minecraftdiamondsword for big CNC_v6 (Autodesk Fusion 360 design; units mm, degrees)
Autodesk Fusion 360 part; units mm, degrees
sketch "big huge diamond sword" plane through (0, 0, 0) normal (0, 0, 1) x (1, 0, 0)
  line L0 (-59.0146, -27.1837) -> (-49.7146, -27.1837)
  line L1 (-49.7146, -27.1837) -> (-49.7146, -17.8837)
  line L2 (-49.7146, -17.8837) -> (-59.0146, -17.8837)
  line L3 (-59.0146, -17.8837) -> (-59.0146, -27.1837)
  line L4 (-49.7146, -27.1837) -> (-40.4146, -27.1837)
  line L5 (-40.4146, -27.1837) -> (-40.4146, -17.8837)
  line L6 (-40.4146, -17.8837) -> (-49.7146, -17.8837)
  line L7 (-49.7146, -17.8837) -> (-49.7146, -27.1837)
  line L8 (-40.4146, -27.1837) -> (-31.1146, -27.1837)
  line L9 (-31.1146, -27.1837) -> (-31.1146, -17.8837)
  line L10 (-40.4146, -17.8837) -> (-40.4146, -27.1837)
  line L11 (-59.0146, -17.8837) -> (-49.7146, -17.8837)
  line L12 (-49.7146, -17.8837) -> (-49.7146, -8.5837)
  line L13 (-49.7146, -8.5837) -> (-59.0146, -8.5837)
  line L14 (-59.0146, -8.5837) -> (-59.0146, -17.8837)
  line L15 (-49.7146, -8.5837) -> (-40.4146, -8.5837)
  line L16 (-40.4146, -8.5837) -> (-40.4146, -17.8837)
  line L17 (-40.4146, -17.8837) -> (-49.7146, -17.8837)
  line L18 (-49.7146, -17.8837) -> (-49.7146, -8.5837)
  line L19 (-59.0146, -8.5837) -> (-49.7146, -8.5837)
  line L20 (-49.7146, -8.5837) -> (-49.7146, 0.7163)
  line L21 (-49.7146, 0.7163) -> (-59.0146, 0.7163)
  line L22 (-59.0146, 0.7163) -> (-59.0146, -8.5837)
  line L23 (-49.7146, -8.5837) -> (-40.4146, -8.5837)
  line L24 (-40.4146, -8.5837) -> (-40.4146, 0.7163)
  line L25 (-40.4146, 0.7163) -> (-49.7146, 0.7163)
  line L26 (-49.7146, 0.7163) -> (-49.7146, -8.5837)
  line L27 (-40.4146, -8.5837) -> (-31.1146, -8.5837)
  line L28 (-31.1146, -8.5837) -> (-31.1146, -17.8837)
  line L29 (-31.1146, -17.8837) -> (-40.4146, -17.8837)
  line L30 (-40.4146, -17.8837) -> (-40.4146, -8.5837)
  line L31 (-40.4146, -8.5837) -> (-31.1146, -8.5837)
  line L32 (-31.1146, -8.5837) -> (-31.1146, 0.7163)
  line L33 (-31.1146, 0.7163) -> (-40.4146, 0.7163)
  line L34 (-40.4146, 0.7163) -> (-40.4146, -8.5837)
  line L35 (-40.4146, 0.7163) -> (-31.1146, 0.7163)
  line L36 (-31.1146, 0.7163) -> (-31.1146, 10.0163)
  line L37 (-31.1146, 10.0163) -> (-40.4146, 10.0163)
  line L38 (-40.4146, 10.0163) -> (-40.4146, 0.7163)
  line L39 (-31.1146, 0.7163) -> (-21.8146, 0.7163)
  line L40 (-21.8146, 0.7163) -> (-21.8146, -8.5837)
  line L41 (-21.8146, -8.5837) -> (-31.1146, -8.5837)
  line L42 (-31.1146, -8.5837) -> (-31.1146, 0.7163)
  line L43 (-31.1146, 0.7163) -> (-21.8146, 0.7163)
  line L44 (-21.8146, 0.7163) -> (-21.8146, 10.0163)
  line L45 (-21.8146, 10.0163) -> (-31.1146, 10.0163)
  line L46 (-31.1146, 10.0163) -> (-31.1146, 0.7163)
  line L47 (-31.1146, 10.0163) -> (-21.8146, 10.0163)
  line L48 (-21.8146, 10.0163) -> (-21.8146, 19.3163)
  line L49 (-21.8146, 19.3163) -> (-31.1146, 19.3163)
  line L50 (-31.1146, 19.3163) -> (-31.1146, 10.0163)
  line L51 (-21.8146, 10.0163) -> (-12.5146, 10.0163)
  line L52 (-12.5146, 0.7163) -> (-21.8146, 0.7163)
  line L53 (-21.8146, 0.7163) -> (-21.8146, 10.0163)
  line L54 (-21.8146, 10.0163) -> (-12.5146, 10.0163)
  line L55 (-12.5146, 10.0163) -> (-12.5146, 19.3163)
  line L56 (-12.5146, 19.3163) -> (-21.8146, 19.3163)
  line L57 (-21.8146, 19.3163) -> (-21.8146, 10.0163)
  line L58 (-21.8146, 19.3163) -> (-12.5146, 19.3163)
  line L59 (-12.5146, 19.3163) -> (-12.5146, 28.6163)
  line L60 (-12.5146, 28.6163) -> (-21.8146, 28.6163)
  line L61 (-21.8146, 28.6163) -> (-21.8146, 19.3163)
  line L62 (-21.8146, 28.6163) -> (-31.1146, 28.6163)
  line L63 (-31.1146, 28.6163) -> (-31.1146, 37.9163)
  line L64 (-31.1146, 37.9163) -> (-21.8146, 37.9163)
  line L65 (-21.8146, 37.9163) -> (-21.8146, 28.6163)
  line L66 (-31.1146, 37.9163) -> (-21.8146, 37.9163)
  line L67 (-21.8146, 37.9163) -> (-21.8146, 47.2163)
  line L68 (-21.8146, 47.2163) -> (-31.1146, 47.2163)
  line L69 (-31.1146, 47.2163) -> (-31.1146, 37.9163)
  line L70 (-31.1146, 47.2163) -> (-40.4146, 47.2163)
  line L71 (-40.4146, 47.2163) -> (-40.4146, 56.5163)
  line L72 (-40.4146, 56.5163) -> (-31.1146, 56.5163)
  line L73 (-31.1146, 56.5163) -> (-31.1146, 47.2163)
  line L74 (-40.4146, 56.5163) -> (-31.1146, 56.5163)
  line L75 (-31.1146, 56.5163) -> (-31.1146, 65.8163)
  line L76 (-31.1146, 65.8163) -> (-40.4146, 65.8163)
  line L77 (-40.4146, 65.8163) -> (-40.4146, 56.5163)
  line L78 (-31.1146, 56.5163) -> (-21.8146, 56.5163)
  line L79 (-21.8146, 56.5163) -> (-21.8146, 65.8163)
  line L80 (-21.8146, 65.8163) -> (-31.1146, 65.8163)
  line L81 (-31.1146, 65.8163) -> (-31.1146, 56.5163)
  line L82 (-31.1146, 47.2163) -> (-21.8146, 47.2163)
  line L83 (-21.8146, 47.2163) -> (-21.8146, 56.5163)
  line L84 (-21.8146, 56.5163) -> (-31.1146, 56.5163)
  line L85 (-31.1146, 56.5163) -> (-31.1146, 47.2163)
  line L86 (-21.8146, 56.5163) -> (-12.5146, 56.5163)
  line L87 (-12.5146, 56.5163) -> (-12.5146, 47.2163)
  line L88 (-12.5146, 47.2163) -> (-21.8146, 47.2163)
  line L89 (-21.8146, 47.2163) -> (-21.8146, 56.5163)
  line L90 (-21.8146, 47.2163) -> (-12.5146, 47.2163)
  line L91 (-12.5146, 47.2163) -> (-12.5146, 37.9163)
  line L92 (-12.5146, 37.9163) -> (-21.8146, 37.9163)
  line L93 (-21.8146, 37.9163) -> (-21.8146, 47.2163)
  line L94 (-21.8146, 28.6163) -> (-12.5146, 28.6163)
  line L95 (-12.5146, 28.6163) -> (-12.5146, 37.9163)
  line L96 (-12.5146, 37.9163) -> (-21.8146, 37.9163)
  line L97 (-21.8146, 37.9163) -> (-21.8146, 28.6163)
  line L98 (-12.5146, 10.0163) -> (-3.2146, 10.0163)
  line L99 (-12.5146, 0.7163) -> (-12.5146, 10.0163)
  line L100 (-12.5146, 19.3163) -> (-3.2146, 19.3163)
  line L101 (-3.2146, 19.3163) -> (-3.2146, 10.0163)
  line L102 (-12.5146, 10.0163) -> (-12.5146, 19.3163)
  line L103 (-12.5146, 28.6163) -> (-3.2146, 28.6163)
  line L104 (-3.2146, 28.6163) -> (-3.2146, 19.3163)
  line L105 (-3.2146, 19.3163) -> (-12.5146, 19.3163)
  line L106 (-12.5146, 19.3163) -> (-12.5146, 28.6163)
  line L107 (-3.2146, 10.0163) -> (6.0854, 10.0163)
  line L108 (6.0854, 10.0163) -> (6.0854, 0.7163)
  line L109 (6.0854, 0.7163) -> (-3.2146, 0.7163)
  line L110 (-3.2146, 0.7163) -> (-3.2146, 10.0163)
  line L111 (-3.2146, 10.0163) -> (6.0854, 10.0163)
  line L112 (6.0854, 10.0163) -> (6.0854, 19.3163)
  line L113 (6.0854, 19.3163) -> (-3.2146, 19.3163)
  line L114 (-3.2146, 19.3163) -> (-3.2146, 10.0163)
  line L115 (6.0854, 10.0163) -> (15.3854, 10.0163)
  line L116 (15.3854, 10.0163) -> (15.3854, 0.7163)
  line L117 (15.3854, 0.7163) -> (6.0854, 0.7163)
  line L118 (6.0854, 0.7163) -> (6.0854, 10.0163)
  line L119 (15.3854, 0.7163) -> (24.6854, 0.7163)
  line L120 (24.6854, 0.7163) -> (24.6854, 10.0163)
  line L121 (24.6854, 10.0163) -> (15.3854, 10.0163)
  line L122 (15.3854, 10.0163) -> (15.3854, 0.7163)
  line L123 (24.6854, 0.7163) -> (33.9854, 0.7163)
  line L124 (33.9854, 0.7163) -> (33.9854, 10.0163)
  line L125 (33.9854, 10.0163) -> (24.6854, 10.0163)
  line L126 (24.6854, 10.0163) -> (24.6854, 0.7163)
  line L127 (15.3854, 0.7163) -> (24.6854, 0.7163)
  line L128 (24.6854, 0.7163) -> (24.6854, -8.5837)
  line L129 (24.6854, -8.5837) -> (15.3854, -8.5837)
  line L130 (15.3854, -8.5837) -> (15.3854, 0.7163)
  line L131 (24.6854, 0.7163) -> (33.9854, 0.7163)
  line L132 (33.9854, 0.7163) -> (33.9854, -8.5837)
  line L133 (33.9854, -8.5837) -> (24.6854, -8.5837)
  line L134 (24.6854, -8.5837) -> (24.6854, 0.7163)
  line L135 (-12.5146, 37.9163) -> (-3.2146, 37.9163)
  line L136 (-3.2146, 37.9163) -> (-3.2146, 28.6163)
  line L137 (-3.2146, 28.6163) -> (-12.5146, 28.6163)
  line L138 (-12.5146, 28.6163) -> (-12.5146, 37.9163)
  line L139 (-3.2146, 28.6163) -> (6.0854, 28.6163)
  line L140 (6.0854, 28.6163) -> (6.0854, 19.3163)
  line L141 (6.0854, 19.3163) -> (-3.2146, 19.3163)
  line L142 (-3.2146, 19.3163) -> (-3.2146, 28.6163)
  line L143 (-12.5146, 47.2163) -> (-3.2146, 47.2163)
  line L144 (-3.2146, 47.2163) -> (-3.2146, 37.9163)
  line L145 (-3.2146, 37.9163) -> (-12.5146, 37.9163)
  line L146 (-12.5146, 37.9163) -> (-12.5146, 47.2163)
  line L147 (-3.2146, 37.9163) -> (6.0854, 37.9163)
  line L148 (6.0854, 37.9163) -> (6.0854, 28.6163)
  line L149 (6.0854, 28.6163) -> (-3.2146, 28.6163)
  line L150 (-3.2146, 28.6163) -> (-3.2146, 37.9163)
  line L151 (-3.2146, 47.2163) -> (6.0854, 47.2163)
  line L152 (6.0854, 47.2163) -> (6.0854, 37.9163)
  line L153 (6.0854, 37.9163) -> (-3.2146, 37.9163)
  line L154 (-3.2146, 37.9163) -> (-3.2146, 47.2163)
  line L155 (6.0854, 19.3163) -> (15.3854, 19.3163)
  line L156 (15.3854, 19.3163) -> (15.3854, 10.0163)
  line L157 (15.3854, 10.0163) -> (6.0854, 10.0163)
  line L158 (6.0854, 10.0163) -> (6.0854, 19.3163)
  line L159 (15.3854, 19.3163) -> (24.6854, 19.3163)
  line L160 (24.6854, 19.3163) -> (24.6854, 10.0163)
  line L161 (24.6854, 10.0163) -> (15.3854, 10.0163)
  line L162 (15.3854, 10.0163) -> (15.3854, 19.3163)
  line L163 (6.0854, 28.6163) -> (15.3854, 28.6163)
  line L164 (15.3854, 28.6163) -> (15.3854, 19.3163)
  line L165 (15.3854, 19.3163) -> (6.0854, 19.3163)
  line L166 (6.0854, 19.3163) -> (6.0854, 28.6163)
  line L167 (6.0854, 37.9163) -> (15.3854, 37.9163)
  line L168 (15.3854, 37.9163) -> (15.3854, 28.6163)
  line L169 (15.3854, 28.6163) -> (6.0854, 28.6163)
  line L170 (6.0854, 28.6163) -> (6.0854, 37.9163)
  line L171 (15.3854, 28.6163) -> (6.0854, 28.6163)
  line L172 (6.0854, 28.6163) -> (6.0854, 37.9163)
  line L173 (6.0854, 37.9163) -> (15.3854, 37.9163)
  line L174 (15.3854, 37.9163) -> (15.3854, 28.6163)
  line L175 (15.3854, 28.6163) -> (24.6854, 28.6163)
  line L176 (24.6854, 28.6163) -> (24.6854, 37.9163)
  line L177 (24.6854, 37.9163) -> (15.3854, 37.9163)
  line L178 (15.3854, 37.9163) -> (15.3854, 28.6163)
  line L179 (6.0854, 37.9163) -> (15.3854, 37.9163)
  line L180 (15.3854, 37.9163) -> (15.3854, 47.2163)
  line L181 (15.3854, 47.2163) -> (6.0854, 47.2163)
  line L182 (6.0854, 47.2163) -> (6.0854, 37.9163)
  line L183 (15.3854, 37.9163) -> (24.6854, 37.9163)
  line L184 (24.6854, 37.9163) -> (24.6854, 47.2163)
  line L185 (24.6854, 47.2163) -> (15.3854, 47.2163)
  line L186 (15.3854, 47.2163) -> (15.3854, 37.9163)
  line L187 (24.6854, 37.9163) -> (33.9854, 37.9163)
  line L188 (33.9854, 37.9163) -> (33.9854, 47.2163)
  line L189 (33.9854, 47.2163) -> (24.6854, 47.2163)
  line L190 (24.6854, 47.2163) -> (24.6854, 37.9163)
  line L191 (-3.2146, 47.2163) -> (6.0854, 47.2163)
  line L192 (6.0854, 47.2163) -> (6.0854, 56.5163)
  line L193 (6.0854, 56.5163) -> (-3.2146, 56.5163)
  line L194 (-3.2146, 56.5163) -> (-3.2146, 47.2163)
  line L195 (6.0854, 47.2163) -> (15.3854, 47.2163)
  line L196 (15.3854, 47.2163) -> (15.3854, 56.5163)
  line L197 (15.3854, 56.5163) -> (6.0854, 56.5163)
  line L198 (6.0854, 56.5163) -> (6.0854, 47.2163)
  line L199 (15.3854, 56.5163) -> (6.0854, 56.5163)
  line L200 (6.0854, 56.5163) -> (6.0854, 65.8163)
  line L201 (6.0854, 65.8163) -> (15.3854, 65.8163)
  line L202 (15.3854, 65.8163) -> (15.3854, 56.5163)
  line L203 (15.3854, 47.2163) -> (24.6854, 47.2163)
  line L204 (24.6854, 47.2163) -> (24.6854, 56.5163)
  line L205 (24.6854, 56.5163) -> (15.3854, 56.5163)
  line L206 (15.3854, 56.5163) -> (15.3854, 47.2163)
  line L207 (15.3854, 56.5163) -> (24.6854, 56.5163)
  line L208 (24.6854, 56.5163) -> (24.6854, 65.8163)
  line L209 (24.6854, 65.8163) -> (15.3854, 65.8163)
  line L210 (15.3854, 65.8163) -> (15.3854, 56.5163)
  line L211 (24.6854, 47.2163) -> (33.9854, 47.2163)
  line L212 (33.9854, 47.2163) -> (33.9854, 56.5163)
  line L213 (33.9854, 56.5163) -> (24.6854, 56.5163)
  line L214 (24.6854, 56.5163) -> (24.6854, 47.2163)
  line L215 (15.3854, 65.8163) -> (24.6854, 65.8163)
  line L216 (24.6854, 65.8163) -> (24.6854, 75.1163)
  line L217 (24.6854, 75.1163) -> (15.3854, 75.1163)
  line L218 (15.3854, 75.1163) -> (15.3854, 65.8163)
  line L219 (33.9854, 47.2163) -> (43.2854, 47.2163)
  line L220 (43.2854, 47.2163) -> (43.2854, 56.5163)
  line L221 (43.2854, 56.5163) -> (33.9854, 56.5163)
  line L222 (33.9854, 56.5163) -> (33.9854, 47.2163)
  line L223 (24.6854, 56.5163) -> (33.9854, 56.5163)
  line L224 (33.9854, 56.5163) -> (33.9854, 65.8163)
  line L225 (33.9854, 65.8163) -> (24.6854, 65.8163)
  line L226 (24.6854, 65.8163) -> (24.6854, 56.5163)
  line L227 (33.9854, 65.8163) -> (43.2854, 65.8163)
  line L228 (43.2854, 65.8163) -> (43.2854, 75.1163)
  line L229 (43.2854, 75.1163) -> (33.9854, 75.1163)
  line L230 (33.9854, 75.1163) -> (33.9854, 65.8163)
  line L231 (33.9854, 65.8163) -> (24.6854, 65.8163)
  line L232 (24.6854, 65.8163) -> (24.6854, 75.1163)
  line L233 (24.6854, 75.1163) -> (33.9854, 75.1163)
  line L234 (33.9854, 75.1163) -> (33.9854, 65.8163)
  line L235 (33.9854, 65.8163) -> (43.2854, 65.8163)
  line L236 (43.2854, 65.8163) -> (43.2854, 56.5163)
  line L237 (43.2854, 56.5163) -> (33.9854, 56.5163)
  line L238 (33.9854, 56.5163) -> (33.9854, 65.8163)
  line L239 (24.6854, 75.1163) -> (33.9854, 75.1163)
  line L240 (33.9854, 75.1163) -> (33.9854, 84.4163)
  line L241 (33.9854, 84.4163) -> (24.6854, 84.4163)
  line L242 (24.6854, 84.4163) -> (24.6854, 75.1163)
  line L243 (33.9854, 75.1163) -> (43.2854, 75.1163)
  line L244 (43.2854, 75.1163) -> (43.2854, 84.4163)
  line L245 (43.2854, 84.4163) -> (33.9854, 84.4163)
  line L246 (33.9854, 84.4163) -> (33.9854, 75.1163)
  line L247 (43.2854, 56.5163) -> (52.5854, 56.5163)
  line L248 (52.5854, 56.5163) -> (52.5854, 65.8163)
  line L249 (52.5854, 65.8163) -> (43.2854, 65.8163)
  line L250 (43.2854, 65.8163) -> (43.2854, 56.5163)
  line L251 (43.2854, 65.8163) -> (52.5854, 65.8163)
  line L252 (52.5854, 65.8163) -> (52.5854, 75.1163)
  line L253 (52.5854, 75.1163) -> (43.2854, 75.1163)
  line L254 (43.2854, 75.1163) -> (43.2854, 65.8163)
  line L255 (43.2854, 75.1163) -> (52.5854, 75.1163)
  line L256 (52.5854, 75.1163) -> (52.5854, 84.4163)
  line L257 (52.5854, 84.4163) -> (43.2854, 84.4163)
  line L258 (43.2854, 84.4163) -> (43.2854, 75.1163)
  line L259 (33.9854, 84.4163) -> (43.2854, 84.4163)
  line L260 (43.2854, 84.4163) -> (43.2854, 93.7163)
  line L261 (43.2854, 93.7163) -> (33.9854, 93.7163)
  line L262 (33.9854, 93.7163) -> (33.9854, 84.4163)
  line L263 (52.5854, 65.8163) -> (61.8854, 65.8163)
  line L264 (61.8854, 65.8163) -> (61.8854, 75.1163)
  line L265 (61.8854, 75.1163) -> (52.5854, 75.1163)
  line L266 (52.5854, 75.1163) -> (52.5854, 65.8163)
  line L267 (43.2854, 84.4163) -> (52.5854, 84.4163)
  line L268 (52.5854, 84.4163) -> (52.5854, 93.7163)
  line L269 (52.5854, 93.7163) -> (43.2854, 93.7163)
  line L270 (43.2854, 93.7163) -> (43.2854, 84.4163)
  line L271 (52.5854, 75.1163) -> (61.8854, 75.1163)
  line L272 (61.8854, 75.1163) -> (61.8854, 84.4163)
  line L273 (61.8854, 84.4163) -> (52.5854, 84.4163)
  line L274 (52.5854, 84.4163) -> (52.5854, 75.1163)
  line L275 (52.5854, 84.4163) -> (61.8854, 84.4163)
  line L276 (61.8854, 84.4163) -> (61.8854, 93.7163)
  line L277 (61.8854, 93.7163) -> (52.5854, 93.7163)
  line L278 (52.5854, 93.7163) -> (52.5854, 84.4163)
  line L279 (61.8854, 75.1163) -> (71.1854, 75.1163)
  line L280 (71.1854, 75.1163) -> (71.1854, 84.4163)
  line L281 (71.1854, 84.4163) -> (61.8854, 84.4163)
  line L282 (61.8854, 84.4163) -> (61.8854, 75.1163)
  line L283 (43.2854, 93.7163) -> (52.5854, 93.7163)
  line L284 (52.5854, 93.7163) -> (52.5854, 103.0163)
  line L285 (52.5854, 103.0163) -> (43.2854, 103.0163)
  line L286 (43.2854, 103.0163) -> (43.2854, 93.7163)
  line L287 (61.8854, 93.7163) -> (71.1854, 93.7163)
  line L288 (71.1854, 93.7163) -> (71.1854, 84.4163)
  line L289 (71.1854, 84.4163) -> (61.8854, 84.4163)
  line L290 (61.8854, 84.4163) -> (61.8854, 93.7163)
  line L291 (52.5854, 93.7163) -> (61.8854, 93.7163)
  line L292 (61.8854, 93.7163) -> (61.8854, 103.0163)
  line L293 (61.8854, 103.0163) -> (52.5854, 103.0163)
  line L294 (52.5854, 103.0163) -> (52.5854, 93.7163)
  line L295 (61.8854, 93.7163) -> (71.1854, 93.7163)
  line L296 (71.1854, 93.7163) -> (71.1854, 103.0163)
  line L297 (71.1854, 103.0163) -> (61.8854, 103.0163)
  line L298 (61.8854, 103.0163) -> (61.8854, 93.7163)
  line L299 (71.1854, 84.4163) -> (80.4854, 84.4163)
  line L300 (80.4854, 84.4163) -> (80.4854, 93.7163)
  line L301 (80.4854, 93.7163) -> (71.1854, 93.7163)
  line L302 (71.1854, 93.7163) -> (71.1854, 84.4163)
  line L303 (52.5854, 103.0163) -> (61.8854, 103.0163)
  line L304 (61.8854, 103.0163) -> (61.8854, 112.3163)
  line L305 (61.8854, 112.3163) -> (52.5854, 112.3163)
  line L306 (52.5854, 112.3163) -> (52.5854, 103.0163)
  line L307 (61.8854, 112.3163) -> (71.1854, 112.3163)
  line L308 (71.1854, 112.3163) -> (71.1854, 103.0163)
  line L309 (71.1854, 103.0163) -> (61.8854, 103.0163)
  line L310 (61.8854, 103.0163) -> (61.8854, 112.3163)
  line L311 (71.1854, 93.7163) -> (80.4854, 93.7163)
  line L312 (80.4854, 93.7163) -> (80.4854, 103.0163)
  line L313 (80.4854, 103.0163) -> (71.1854, 103.0163)
  line L314 (71.1854, 103.0163) -> (71.1854, 93.7163)
  line L315 (71.1854, 103.0163) -> (80.4854, 103.0163)
  line L316 (80.4854, 103.0163) -> (80.4854, 112.3163)
  line L317 (80.4854, 112.3163) -> (71.1854, 112.3163)
  line L318 (71.1854, 112.3163) -> (71.1854, 103.0163)
  line L319 (61.8854, 112.3163) -> (71.1854, 112.3163)
  line L320 (71.1854, 112.3163) -> (71.1854, 121.6163)
  line L321 (71.1854, 121.6163) -> (61.8854, 121.6163)
  line L322 (61.8854, 121.6163) -> (61.8854, 112.3163)
  line L323 (71.1854, 112.3163) -> (80.4854, 112.3163)
  line L324 (80.4854, 112.3163) -> (80.4854, 121.6163)
  line L325 (80.4854, 121.6163) -> (71.1854, 121.6163)
  line L326 (71.1854, 121.6163) -> (71.1854, 112.3163)
  line L327 (80.4854, 93.7163) -> (89.7854, 93.7163)
  line L328 (89.7854, 93.7163) -> (89.7854, 103.0163)
  line L329 (89.7854, 103.0163) -> (80.4854, 103.0163)
  line L330 (80.4854, 103.0163) -> (80.4854, 93.7163)
  line L331 (80.4854, 103.0163) -> (89.7854, 103.0163)
  line L332 (89.7854, 103.0163) -> (89.7854, 112.3163)
  line L333 (89.7854, 112.3163) -> (80.4854, 112.3163)
  line L334 (80.4854, 112.3163) -> (80.4854, 103.0163)
  line L335 (80.4854, 112.3163) -> (71.1854, 112.3163)
  line L336 (71.1854, 112.3163) -> (71.1854, 121.6163)
  line L337 (71.1854, 121.6163) -> (80.4854, 121.6163)
  line L338 (80.4854, 121.6163) -> (80.4854, 112.3163)
  line L339 (80.4854, 112.3163) -> (89.7854, 112.3163)
  line L340 (89.7854, 112.3163) -> (89.7854, 121.6163)
  line L341 (89.7854, 121.6163) -> (80.4854, 121.6163)
  line L342 (80.4854, 121.6163) -> (80.4854, 112.3163)
  dimension "d249" = 9.3
  dimension "d250" = 9.3
  dimension "d251" = 9.3
  dimension "d252" = 9.3
  dimension "d253" = 9.3
  dimension "d254" = 9.3
  dimension "d255" = 9.3
  dimension "d256" = 9.3
  dimension "d261" = 9.3
  dimension "d262" = 9.3
  dimension "d263" = 9.3
  dimension "d264" = 9.3
  dimension "d265" = 9.3
  dimension "d266" = 9.3
  dimension "d267" = 9.3
  dimension "d268" = 9.3
  dimension "d271" = 9.3
  dimension "d272" = 9.3
  dimension "d273" = 9.3
  dimension "d274" = 9.3
  dimension "d275" = 9.3
  dimension "d276" = 9.3
  dimension "d277" = 9.3
  dimension "d278" = 9.3
  dimension "d279" = 9.3
  dimension "d280" = 9.3
  dimension "d281" = 9.3
  dimension "d282" = 9.3
  dimension "d283" = 9.3
  dimension "d284" = 9.3
  dimension "d285" = 9.3
  dimension "d286" = 9.3
  dimension "d287" = 9.3
  dimension "d288" = 9.3
  dimension "d289" = 9.3
  dimension "d290" = 9.3
  dimension "d291" = 9.3
  dimension "d292" = 9.3
  dimension "d293" = 9.3
  dimension "d294" = 9.3
  dimension "d295" = 9.3
  dimension "d296" = 9.3
  dimension "d297" = 9.3
  dimension "d298" = 9.3
  dimension "d299" = 9.3
  dimension "d300" = 9.3
  dimension "d301" = 9.3
  dimension "d302" = 9.3
  dimension "d303" = 9.3
  dimension "d304" = 9.3
  dimension "d309" = 9.3
  dimension "d310" = 9.3
  dimension "d311" = 9.3
  dimension "d312" = 9.3
  dimension "d313" = 9.3
  dimension "d314" = 9.3
  dimension "d315" = 9.3
  dimension "d316" = 9.3
  dimension "d319" = 9.3
  dimension "d320" = 9.3
  dimension "d321" = 9.3
  dimension "d322" = 9.3
  dimension "d323" = 9.3
  dimension "d324" = 9.3
  dimension "d325" = 9.3
  dimension "d326" = 9.3
  dimension "d327" = 9.3
  dimension "d328" = 9.3
  dimension "d329" = 9.3
  dimension "d330" = 9.3
  dimension "d331" = 9.3
  dimension "d332" = 9.3
  dimension "d333" = 9.3
  dimension "d334" = 9.3
  dimension "d335" = 9.3
  dimension "d336" = 9.3
  dimension "d337" = 9.3
  dimension "d338" = 9.3
  dimension "d339" = 9.3
  dimension "d340" = 9.3
  dimension "d341" = 9.3
  dimension "d342" = 9.3
  dimension "d343" = 9.3
  dimension "d344" = 9.3
  dimension "d345" = 9.3
  dimension "d346" = 9.3
  dimension "d347" = 9.3
  dimension "d348" = 9.3
  dimension "d349" = 9.3
  dimension "d350" = 9.3
  dimension "d351" = 9.3
  dimension "d352" = 9.3
  dimension "d353" = 9.3
  dimension "d354" = 9.3
  dimension "d355" = 9.3
  dimension "d356" = 9.3
  dimension "d357" = 9.3
  dimension "d358" = 9.3
  dimension "d359" = 9.3
  dimension "d360" = 9.3
  dimension "d361" = 9.3
  dimension "d362" = 9.3
  dimension "d363" = 9.3
  dimension "d364" = 9.3
  dimension "d365" = 9.3
  dimension "d366" = 9.3
  dimension "d367" = 9.3
  dimension "d368" = 9.3
  dimension "d369" = 9.3
  dimension "d370" = 9.3
  dimension "d371" = 9.3
  dimension "d372" = 9.3
  dimension "d373" = 9.3
  dimension "d374" = 9.3
  dimension "d375" = 9.3
  dimension "d376" = 9.3
  dimension "d377" = 9.3
  dimension "d378" = 9.3
  dimension "d379" = 9.3
  dimension "d380" = 9.3
  dimension "d381" = 9.3
  dimension "d382" = 9.3
  dimension "d383" = 9.3
  dimension "d384" = 9.3
  dimension "d385" = 9.3
  dimension "d386" = 9.3
  dimension "d387" = 9.3
  dimension "d388" = 9.3
  dimension "d389" = 9.3
  dimension "d390" = 9.3
  dimension "d391" = 9.3
  dimension "d392" = 9.3
  dimension "d393" = 9.3
  dimension "d394" = 9.3
  dimension "d395" = 9.3
  dimension "d396" = 9.3
  dimension "d397" = 9.3
  dimension "d398" = 9.3
  dimension "d399" = 9.3
  dimension "d400" = 9.3
  dimension "d401" = 9.3
  dimension "d402" = 9.3
  dimension "d403" = 9.3
  dimension "d404" = 9.3
  dimension "d405" = 9.3
  dimension "d406" = 9.3
  dimension "d407" = 9.3
  dimension "d408" = 9.3
  dimension "d409" = 9.3
  dimension "d410" = 9.3
  dimension "d411" = 9.3
  dimension "d412" = 9.3
  dimension "d413" = 9.3
  dimension "d414" = 9.3
  dimension "d415" = 9.3
  dimension "d416" = 9.3
  dimension "d417" = 9.3
  dimension "d418" = 9.3
  dimension "d419" = 9.3
  dimension "d420" = 9.3
  dimension "d421" = 9.3
  dimension "d422" = 9.3
  dimension "d423" = 9.3
  dimension "d424" = 9.3
  dimension "d425" = 9.3
  dimension "d426" = 9.3
  dimension "d427" = 9.3
  dimension "d428" = 9.3
  dimension "d429" = 9.3
  dimension "d430" = 9.3
  dimension "d431" = 9.3
  dimension "d432" = 9.3
  dimension "d433" = 9.3
  dimension "d434" = 9.3
  constraint horizontal L0
  constraint vertical L1
  constraint horizontal L2
  constraint vertical L3
  constraint horizontal L4
  constraint vertical L5
  constraint horizontal L6
  constraint vertical L7
  constraint horizontal L8
  constraint vertical L9
  constraint vertical L10
  constraint horizontal L11
  constraint vertical L12
  constraint horizontal L13
  constraint vertical L14
  constraint horizontal L15
  constraint vertical L16
  constraint horizontal L17
  constraint vertical L18
  constraint horizontal L19
  constraint vertical L20
  constraint horizontal L21
  constraint vertical L22
  constraint horizontal L23
  constraint vertical L24
  constraint horizontal L25
  constraint vertical L26
  constraint horizontal L27
  constraint vertical L28
  constraint horizontal L29
  constraint vertical L30
  constraint horizontal L31
  constraint vertical L32
  constraint horizontal L33
  constraint vertical L34
  constraint horizontal L35
  constraint vertical L36
  constraint horizontal L37
  constraint vertical L38
  constraint horizontal L39
  constraint vertical L40
  constraint horizontal L41
  constraint vertical L42
  constraint horizontal L43
  constraint vertical L44
  constraint horizontal L45
  constraint vertical L46
  constraint horizontal L47
  constraint vertical L48
  constraint horizontal L49
  constraint vertical L50
  constraint horizontal L51
  constraint horizontal L52
  constraint vertical L53
  constraint horizontal L54
  constraint vertical L55
  constraint horizontal L56
  constraint vertical L57
  constraint horizontal L58
  constraint vertical L59
  constraint horizontal L60
  constraint vertical L61
  constraint horizontal L62
  constraint vertical L63
  constraint horizontal L64
  constraint vertical L65
  constraint horizontal L66
  constraint vertical L67
  constraint horizontal L68
  constraint vertical L69
  constraint horizontal L70
  constraint vertical L71
  constraint horizontal L72
  constraint vertical L73
  constraint vertical L75
  constraint perpendicular L74 L75
  constraint horizontal L76
  constraint parallel L75 L77
  constraint vertical L79
  constraint perpendicular L78 L79
  constraint horizontal L80
  constraint parallel L79 L81
  constraint horizontal L82
  constraint vertical L83
  constraint horizontal L84
  constraint vertical L85
  constraint vertical L87
  constraint perpendicular L86 L87
  constraint horizontal L88
  constraint parallel L87 L89
  constraint horizontal L90
  constraint vertical L91
  constraint horizontal L92
  constraint vertical L93
  constraint horizontal L94
  constraint vertical L95
  constraint horizontal L96
  constraint vertical L97
  constraint horizontal L100
  constraint vertical L101
  constraint vertical L102
  constraint vertical L104
  constraint perpendicular L103 L104
  constraint horizontal L105
  constraint parallel L104 L106
  constraint horizontal L107
  constraint vertical L108
  constraint horizontal L109
  constraint vertical L110
  constraint perpendicular L52 L99
  constraint horizontal L98
  constraint coincident L98.end L101.end
  constraint horizontal L111
  constraint vertical L112
  constraint horizontal L113
  constraint vertical L114
  constraint vertical L116
  constraint perpendicular L115 L116
  constraint horizontal L117
  constraint parallel L116 L118
  constraint horizontal L119
  constraint vertical L120
  constraint horizontal L121
  constraint vertical L122
  constraint vertical L124
  constraint perpendicular L123 L124
  constraint horizontal L125
  constraint parallel L124 L126
  constraint vertical L128
  constraint perpendicular L127 L128
  constraint horizontal L129
  constraint parallel L128 L130
  constraint vertical L132
  constraint perpendicular L131 L132
  constraint horizontal L133
  constraint parallel L132 L134
  constraint vertical L136
  constraint perpendicular L135 L136
  constraint horizontal L137
  constraint parallel L136 L138
  constraint vertical L140
  constraint perpendicular L139 L140
  constraint horizontal L141
  constraint parallel L140 L142
  constraint vertical L144
  constraint perpendicular L143 L144
  constraint horizontal L145
  constraint parallel L144 L146
  constraint vertical L148
  constraint perpendicular L147 L148
  constraint horizontal L149
  constraint parallel L148 L150
  constraint vertical L152
  constraint perpendicular L151 L152
  constraint horizontal L153
  constraint parallel L152 L154
  constraint vertical L156
  constraint perpendicular L155 L156
  constraint horizontal L157
  constraint parallel L156 L158
  constraint vertical L160
  constraint perpendicular L159 L160
  constraint horizontal L161
  constraint parallel L160 L162
  constraint vertical L164
  constraint perpendicular L163 L164
  constraint horizontal L165
  constraint parallel L164 L166
  constraint vertical L168
  constraint perpendicular L167 L168
  constraint horizontal L169
  constraint parallel L168 L170
  constraint vertical L172
  constraint perpendicular L171 L172
  constraint horizontal L173
  constraint parallel L172 L174
  constraint vertical L176
  constraint perpendicular L175 L176
  constraint horizontal L177
  constraint parallel L176 L178
  constraint vertical L180
  constraint perpendicular L179 L180
  constraint horizontal L181
  constraint parallel L180 L182
  constraint vertical L184
  constraint perpendicular L183 L184
  constraint horizontal L185
  constraint parallel L184 L186
  constraint vertical L188
  constraint perpendicular L187 L188
  constraint horizontal L189
  constraint parallel L188 L190
  constraint horizontal L191
  constraint vertical L192
  constraint horizontal L193
  constraint vertical L194
  constraint vertical L196
  constraint perpendicular L195 L196
  constraint horizontal L197
  constraint parallel L196 L198
  constraint vertical L200
  constraint perpendicular L199 L200
  constraint horizontal L201
  constraint parallel L200 L202
  constraint vertical L204
  constraint perpendicular L203 L204
  constraint horizontal L205
  constraint parallel L204 L206
  constraint horizontal L207
  constraint vertical L208
  constraint horizontal L209
  constraint vertical L210
  constraint vertical L212
  constraint perpendicular L211 L212
  constraint horizontal L213
  constraint parallel L212 L214
  constraint vertical L216
  constraint perpendicular L215 L216
  constraint horizontal L217
  constraint parallel L216 L218
  constraint vertical L220
  constraint perpendicular L219 L220
  constraint horizontal L221
  constraint parallel L220 L222
  constraint vertical L224
  constraint perpendicular L223 L224
  constraint horizontal L225
  constraint parallel L224 L226
  constraint vertical L228
  constraint perpendicular L227 L228
  constraint horizontal L229
  constraint parallel L228 L230
  constraint vertical L232
  constraint perpendicular L231 L232
  constraint horizontal L233
  constraint parallel L232 L234
  constraint vertical L236
  constraint perpendicular L235 L236
  constraint horizontal L237
  constraint parallel L236 L238
  constraint vertical L240
  constraint perpendicular L239 L240
  constraint horizontal L241
  constraint parallel L240 L242
  constraint vertical L244
  constraint perpendicular L243 L244
  constraint horizontal L245
  constraint parallel L244 L246
  constraint vertical L248
  constraint perpendicular L247 L248
  constraint horizontal L249
  constraint parallel L248 L250
  constraint vertical L252
  constraint perpendicular L251 L252
  constraint horizontal L253
  constraint parallel L252 L254
  constraint vertical L256
  constraint perpendicular L255 L256
  constraint horizontal L257
  constraint parallel L256 L258
  constraint vertical L260
  constraint perpendicular L259 L260
  constraint horizontal L261
  constraint parallel L260 L262
  constraint vertical L264
  constraint perpendicular L263 L264
  constraint horizontal L265
  constraint parallel L264 L266
  constraint vertical L268
  constraint perpendicular L267 L268
  constraint horizontal L269
  constraint parallel L268 L270
  constraint horizontal L271
  constraint vertical L272
  constraint horizontal L273
  constraint vertical L274
  constraint vertical L276
  constraint perpendicular L275 L276
  constraint horizontal L277
  constraint parallel L276 L278
  constraint vertical L280
  constraint perpendicular L279 L280
  constraint horizontal L281
  constraint parallel L280 L282
  constraint vertical L284
  constraint perpendicular L283 L284
  constraint horizontal L285
  constraint parallel L284 L286
  constraint vertical L288
  constraint perpendicular L287 L288
  constraint horizontal L289
  constraint parallel L288 L290
  constraint vertical L292
  constraint perpendicular L291 L292
  constraint horizontal L293
  constraint parallel L292 L294
  constraint horizontal L295
  constraint vertical L296
  constraint horizontal L297
  constraint vertical L298
  constraint horizontal L299
  constraint vertical L300
  constraint horizontal L301
  constraint vertical L302
  constraint vertical L304
  constraint perpendicular L303 L304
  constraint horizontal L305
  constraint parallel L304 L306
  constraint horizontal L307
  constraint vertical L308
  constraint horizontal L309
  constraint vertical L310
  constraint horizontal L311
  constraint vertical L312
  constraint horizontal L313
  constraint vertical L314
  constraint horizontal L315
  constraint vertical L316
  constraint horizontal L317
  constraint vertical L318
  constraint horizontal L319
  constraint vertical L320
  constraint horizontal L321
  constraint vertical L322
  constraint horizontal L323
  constraint vertical L324
  constraint horizontal L325
  constraint vertical L326
  constraint horizontal L327
  constraint vertical L328
  constraint horizontal L329
  constraint vertical L330
  constraint horizontal L331
  constraint vertical L332
  constraint horizontal L333
  constraint vertical L334
  constraint horizontal L335
  constraint vertical L336
  constraint horizontal L337
  constraint vertical L338
  constraint vertical L340
  constraint perpendicular L339 L340
  constraint horizontal L341
  constraint parallel L340 L342
  measures "d249" distance of L0.start L0.end
  measures "d250" distance of L0.start L2.end
  measures "d251" distance of L0.end L4.end
  measures "d252" distance of L0.end L1.end
  measures "d253" distance of L4.end L8.end
  measures "d254" distance of L4.end L5.end
  measures "d255" distance of L2.end L1.end
  measures "d256" distance of L2.end L13.end
  measures "d261" distance of L12.end L15.end
  measures "d262" distance of L12.end L1.end
  measures "d263" distance of L13.end L12.end
  measures "d264" distance of L13.end L21.end
  measures "d265" distance of L12.end L15.end
  measures "d266" distance of L12.end L20.end
  measures "d267" distance of L15.end L27.end
  measures "d268" distance of L15.end L5.end
  measures "d271" distance of L15.end L27.end
  measures "d272" distance of L15.end L24.end
  measures "d273" distance of L24.end L32.end
  measures "d274" distance of L24.end L37.end
  measures "d275" distance of L32.end L39.end
  measures "d276" distance of L32.end L27.end
  measures "d277" distance of L32.end L39.end
  measures "d278" distance of L32.end L36.end
  measures "d279" distance of L36.end L44.end
  measures "d280" distance of L36.end L49.end
  measures "d281" distance of L44.end L51.end
  measures "d282" distance of L44.end L39.end
  measures "d283" distance of L44.end L51.end
  measures "d284" distance of L44.end L48.end
  measures "d285" distance of L48.end L55.end
  measures "d286" distance of L48.end L60.end
  measures "d287" distance of L60.end L62.end
  measures "d288" distance of L60.end L64.end
  measures "d289" distance of L63.end L64.end
  measures "d290" distance of L63.end L68.end
  measures "d291" distance of L68.end L70.end
  measures "d292" distance of L68.end L72.end
  measures "d293" distance of L71.end L72.end
  measures "d294" distance of L71.end L76.end
  measures "d295" distance of L72.end L78.end
  measures "d296" distance of L72.end L75.end
  measures "d297" distance of L68.end L67.end
  measures "d298" distance of L68.end L72.end
  measures "d299" distance of L78.end L86.end
  measures "d300" distance of L78.end L67.end
  measures "d301" distance of L67.end L87.end
  measures "d302" distance of L67.end L64.end
  measures "d303" distance of L60.end L59.end
  measures "d304" distance of L60.end L64.end
  measures "d309" distance of L51.end L98.end
  measures "d310" distance of L51.end L52.start
  measures "d311" distance of L55.end L100.end
  measures "d312" distance of L55.end L51.end
  measures "d313" distance of L59.end L103.end
  measures "d314" distance of L59.end L55.end
  measures "d315" distance of L98.end L107.end
  measures "d316" distance of L98.end L109.end
  measures "d319" distance of L98.end L107.end
  measures "d320" distance of L98.end L100.end
  measures "d321" distance of L107.end L115.end
  measures "d322" distance of L107.end L108.end
  measures "d323" distance of L116.end L119.end
  measures "d324" distance of L116.end L115.end
  measures "d325" distance of L119.end L123.end
  measures "d326" distance of L119.end L120.end
  measures "d327" distance of L116.end L119.end
  measures "d328" distance of L116.end L129.end
  measures "d329" distance of L119.end L123.end
  measures "d330" distance of L119.end L128.end
  measures "d331" distance of L91.end L135.end
  measures "d332" distance of L91.end L59.end
  measures "d333" distance of L103.end L139.end
  measures "d334" distance of L103.end L100.end
  measures "d335" distance of L87.end L143.end
  measures "d336" distance of L87.end L91.end
  measures "d337" distance of L135.end L147.end
  measures "d338" distance of L135.end L103.end
  measures "d339" distance of L143.end L151.end
  measures "d340" distance of L143.end L135.end
  measures "d341" distance of L112.end L155.end
  measures "d342" distance of L112.end L107.end
  measures "d343" distance of L155.end L159.end
  measures "d344" distance of L155.end L115.end
  measures "d345" distance of L139.end L163.end
  measures "d346" distance of L139.end L112.end
  measures "d347" distance of L147.end L167.end
  measures "d348" distance of L147.end L139.end
  measures "d349" distance of L163.end L139.end
  measures "d350" distance of L163.end L167.end
  measures "d351" distance of L163.end L175.end
  measures "d352" distance of L163.end L167.end
  measures "d353" distance of L147.end L167.end
  measures "d354" distance of L147.end L151.end
  measures "d355" distance of L167.end L176.end
  measures "d356" distance of L167.end L180.end
  measures "d357" distance of L176.end L187.end
  measures "d358" distance of L176.end L184.end
  measures "d359" distance of L143.end L151.end
  measures "d360" distance of L143.end L193.end
  measures "d361" distance of L151.end L180.end
  measures "d362" distance of L151.end L192.end
  measures "d363" distance of L196.end L192.end
  measures "d364" distance of L196.end L201.end
  measures "d365" distance of L180.end L184.end
  measures "d366" distance of L180.end L196.end
  measures "d367" distance of L196.end L204.end
  measures "d368" distance of L196.end L201.end
  measures "d369" distance of L184.end L188.end
  measures "d370" distance of L184.end L204.end
  measures "d371" distance of L201.end L208.end
  measures "d372" distance of L201.end L217.end
  measures "d373" distance of L188.end L219.end
  measures "d374" distance of L188.end L212.end
  measures "d375" distance of L204.end L212.end
  measures "d376" distance of L204.end L208.end
  measures "d377" distance of L224.end L227.end
  measures "d378" distance of L224.end L229.end
  measures "d379" distance of L224.end L208.end
  measures "d380" distance of L224.end L229.end
  measures "d381" distance of L224.end L227.end
  measures "d382" distance of L224.end L212.end
  measures "d383" distance of L216.end L229.end
  measures "d384" distance of L216.end L241.end
  measures "d385" distance of L229.end L228.end
  measures "d386" distance of L229.end L240.end
  measures "d387" distance of L220.end L247.end
  measures "d388" distance of L220.end L227.end
  measures "d389" distance of L227.end L248.end
  measures "d390" distance of L227.end L228.end
  measures "d391" distance of L228.end L252.end
  measures "d392" distance of L228.end L244.end
  measures "d393" distance of L240.end L244.end
  measures "d394" distance of L240.end L261.end
  measures "d395" distance of L248.end L263.end
  measures "d396" distance of L248.end L252.end
  measures "d397" distance of L244.end L256.end
  measures "d398" distance of L244.end L260.end
  measures "d399" distance of L252.end L264.end
  measures "d400" distance of L252.end L256.end
  measures "d401" distance of L256.end L272.end
  measures "d402" distance of L256.end L268.end
  measures "d403" distance of L264.end L279.end
  measures "d404" distance of L264.end L272.end
  measures "d405" distance of L260.end L268.end
  measures "d406" distance of L260.end L285.end
  measures "d407" distance of L276.end L287.end
  measures "d408" distance of L276.end L272.end
  measures "d409" distance of L268.end L276.end
  measures "d410" distance of L268.end L284.end
  measures "d411" distance of L276.end L287.end
  measures "d412" distance of L276.end L292.end
  measures "d413" distance of L280.end L299.end
  measures "d414" distance of L280.end L287.end
  measures "d415" distance of L284.end L292.end
  measures "d416" distance of L284.end L305.end
  measures "d417" distance of L304.end L307.end
  measures "d418" distance of L304.end L292.end
  measures "d419" distance of L287.end L300.end
  measures "d420" distance of L287.end L296.end
  measures "d421" distance of L296.end L312.end
  measures "d422" distance of L296.end L307.end
  measures "d423" distance of L304.end L307.end
  measures "d424" distance of L304.end L321.end
  measures "d425" distance of L307.end L316.end
  measures "d426" distance of L307.end L320.end
  measures "d427" distance of L300.end L327.end
  measures "d428" distance of L300.end L312.end
  measures "d429" distance of L312.end L328.end
  measures "d430" distance of L312.end L316.end
  measures "d431" distance of L316.end L307.end
  measures "d432" distance of L316.end L324.end
  measures "d433" distance of L316.end L332.end
  measures "d434" distance of L316.end L324.end
extrude "Extrude11" add sketch "big huge diamond sword" along normal blind 23 makes body 1
sketch "board prepare" plane through (0, 0, 0) normal (0, 0, 1) x (1, 0, 0)
  line L0 (0, 0) -> (310, 0)
  line L1 (310, 0) -> (310, 124)
  line L2 (310, 124) -> (0, 124)
  line L3 (0, 124) -> (0, 0)
  dimension "d437" = 310
  dimension "d438" = 124
  constraint horizontal L0
  constraint vertical L1
  constraint horizontal L2
  constraint vertical L3
  constraint coincident L0.start L3.end
  measures "d437" distance of L0.start L0.end
  measures "d438" distance of L0.start L2.end
extrude "Extrude12" add sketch "board prepare" along normal blind 25 separate body makes body 2
move_body "Move2" bodies 1 to x (0.707107, -0.707107, 0) y (0.707107, 0.707107, 0) z (0, 0, 1) at (0, 0, 0)
move_body "Move3" bodies 1 to x (1, 0, 0) y (0, 1, 0) z (0, 0, 1) at (136.2, 74.374, -13.1911)
move_body "Move4" bodies 1 to x (1, 0, 0) y (0, 1, 0) z (0, 0, 1) at (-19.8307, -44.2731, -19.9999)
move_body "Move5" bodies 1 to x (1, 0, 0) y (0, 1, 0) z (0, 0, 1) at (-55.4179, 0.0003, 0)
move_body "Move6" bodies 1 to x (1, 0, 0) y (0, 1, 0) z (0, 0, 1) at (0, 0, 33.191)
equation "d = 9.3 mm"
equation "StockHeight = 23 mm"
equation "d249 = d"
equation "d250 = d"
equation "d251 = d"
equation "d252 = d"
equation "d253 = d"
equation "d254 = d"
equation "d255 = d"
equation "d256 = d"
equation "d261 = d"
equation "d262 = d"
equation "d263 = d"
equation "d264 = d"
equation "d265 = d"
equation "d266 = d"
equation "d267 = d"
equation "d268 = d"
equation "d271 = d"
equation "d272 = d"
equation "d273 = d"
equation "d274 = d"
equation "d275 = d"
equation "d276 = d"
equation "d277 = d"
equation "d278 = d"
equation "d279 = d"
equation "d280 = d"
equation "d281 = d"
equation "d282 = d"
equation "d283 = d"
equation "d284 = d"
equation "d285 = d"
equation "d286 = d"
equation "d287 = d"
equation "d288 = d"
equation "d289 = d"
equation "d290 = d"
equation "d291 = d"
equation "d292 = d"
equation "d293 = d"
equation "d294 = d"
equation "d295 = d"
equation "d296 = d"
equation "d297 = d"
equation "d298 = d"
equation "d299 = d"
equation "d300 = d"
equation "d301 = d"
equation "d302 = d"
equation "d303 = d"
equation "d304 = d"
equation "d309 = d"
equation "d310 = d"
equation "d311 = d"
equation "d312 = d"
equation "d313 = d"
equation "d314 = d"
equation "d315 = d"
equation "d316 = d"
equation "d319 = d"
equation "d320 = d"
equation "d321 = d"
equation "d322 = d"
equation "d323 = d"
equation "d324 = d"
equation "d325 = d"
equation "d326 = d"
equation "d327 = d"
equation "d328 = d"
equation "d329 = d"
equation "d330 = d"
equation "d331 = d"
equation "d332 = d"
equation "d333 = d"
equation "d334 = d"
equation "d335 = d"
equation "d336 = d"
equation "d337 = d"
equation "d338 = d"
equation "d339 = d"
equation "d340 = d"
equation "d341 = d"
equation "d342 = d"
equation "d343 = d"
equation "d344 = d"
equation "d345 = d"
equation "d346 = d"
equation "d347 = d"
equation "d348 = d"
equation "d349 = d"
equation "d350 = d"
equation "d351 = d"
equation "d352 = d"
equation "d353 = d"
equation "d354 = d"
equation "d355 = d"
equation "d356 = d"
equation "d357 = d"
equation "d358 = d"
equation "d359 = d"
equation "d360 = d"
equation "d361 = d"
equation "d362 = d"
equation "d363 = d"
equation "d364 = d"
equation "d365 = d"
equation "d366 = d"
equation "d367 = d"
equation "d368 = d"
equation "d369 = d"
equation "d370 = d"
equation "d371 = d"
equation "d372 = d"
equation "d373 = d"
equation "d374 = d"
equation "d375 = d"
equation "d376 = d"
equation "d377 = d"
equation "d378 = d"
equation "d379 = d"
equation "d380 = d"
equation "d381 = d"
equation "d382 = d"
equation "d383 = d"
equation "d384 = d"
equation "d385 = d"
equation "d386 = d"
equation "d387 = d"
equation "d388 = d"
equation "d389 = d"
equation "d390 = d"
equation "d391 = d"
equation "d392 = d"
equation "d393 = d"
equation "d394 = d"
equation "d395 = d"
equation "d396 = d"
equation "d397 = d"
equation "d398 = d"
equation "d399 = d"
equation "d400 = d"
equation "d401 = d"
equation "d402 = d"
equation "d403 = d"
equation "d404 = d"
equation "d405 = d"
equation "d406 = d"
equation "d407 = d"
equation "d408 = d"
equation "d409 = d"
equation "d410 = d"
equation "d411 = d"
equation "d412 = d"
equation "d413 = d"
equation "d414 = d"
equation "d415 = d"
equation "d416 = d"
equation "d417 = d"
equation "d418 = d"
equation "d419 = d"
equation "d420 = d"
equation "d421 = d"
equation "d422 = d"
equation "d423 = d"
equation "d424 = d"
equation "d425 = d"
equation "d426 = d"
equation "d427 = d"
equation "d428 = d"
equation "d429 = d"
equation "d430 = d"
equation "d431 = d"
equation "d432 = d"
equation "d433 = d"
equation "d434 = d"
equation "d435 = StockHeight"
named bodies: "diamond sword body", "board"
